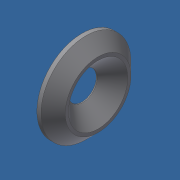
# Autodesk Inventor part: SN213912_M3
Saved by Autodesk Inventor 2021 (Build 250183000, 183)
## iProperties
Created: 2020-11-18
Part Number: SN213912_M3
Material: Acier zingué-bleu
Description: Rondelle pour vis t co
Document SubType Name: Modeling
Designer: Jean-Marc.VULLIAMY
Authority: BN1277
Density: 7.8 g/cm^3
Appearance: Par défaut
Material number: ---
Author: JVY
Autodesk Inventor part; units mm, degrees
ref_plane "Plan YZ" through (0, 0, 0) normal (1, 0, 0) x (0, 1, 0)
ref_plane "Plan XZ" through (0, 0, 0) normal (0, 1, 0) x (-1, 0, 0)
ref_plane "Plan XY" through (0, 0, 0) normal (0, 0, 1) x (1, 0, 0)
sketch "Esquisse1" plane through (0, 0, 0) normal (0, 0, 1) x (1, 0, 0)
  line L0 (0, 5) -> (0, 1.6)
  line L1 (0, 1.6) -> (0.1, 1.6)
  line L2 (0.1, 1.6) -> (1.8, 3.3)
  line L3 (1.8, 3.3) -> (1.8, 3.65)
  line L4 (1.8, 3.65) -> (0.45, 5)
  line L5 (0.45, 5) -> (0, 5)
  line L6 (-2.9261, 0) -> (4.3316, 0) construction
  point P0 (0, 0)
  dimension "d0" = 3.2
  dimension "d1" = 10
  dimension "d2" = 7.3
  dimension "d3" = 6.6
  dimension "d4" = 1.8
  dimension "d5" = 45
  constraints: 14 end point, 3 perpendicular, 2 point on line, 1 horizontal, 1 parallel, 1 vertical
  measures "d0" diameter of L1 L6
  measures "d1" diameter of L5 L6
  measures "d2" diameter of L3.end L6
  measures "d3" diameter of L2.end L6
  measures "d4" distance between parallel lines of L3 L0
  measures "d5" angle of L0 L2
revolve "Révolution1" add sketch "Esquisse1" angle 360 about axis through (-2.9261, 0, 0) along (1, 0, 0)
